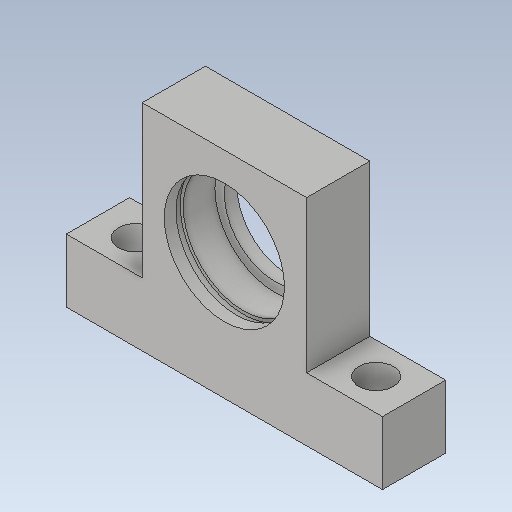
# Autodesk Inventor part: BGHK6800VV-20_h
Saved by Autodesk Inventor 2020.2 (Build 242310000, 310)
## iProperties
Created: 2022-11-02
Part Number: BGHK6800VV-20_h
Material: Generic
Catalog Web Link: www.cadenas.de
Description: BGHKB, BGHK, BGHKA, BGHKSA, BGHKS_housing-Bearings with Housings - T-Shaped - h Selectable
Vendor: MISUMI
Document SubType Name: Modeling
Designer: psAdmin
Manufacturer: MISUMI
Mass: 8.05926 g
Surface Area: 44.1935 cm^2
Volume: 8.05926 cm^3
Density: 1 g/cm^3
Appearance: PSOLRGB-175-175-175
Category: PARTsolutions
Company: MISUMI
PSOL_IDENT_0: {$CADENAS_DATA/23d-libs/misumi/metric/12_bearing_holders/bghkb/bghkb_housing.prj},237 {VTYP=3D},{NB=
PSOL_IDENT_1: BGHK6800VV-20_h},{LINA=BGHK6800VV-20},{NN=BGHKB, BGHK, BGHKA, BGHKSA, BGHKS_housing},{DATE=30.03.201
PSOL_IDENT_2: 8 01:48:21},{GEOMDATE=23.03.2015 00:00:00},{VERSION=},{LINEID=300},{WBVAR=MATB,MATH,STH,SEAL,HH,ALT1
PSOL_IDENT_3: ,ALT2},{WBNUMERIC=HH}  {NB=BGHK6800VV-20_h},{LINA=BGHK6800VV-20},{KT=DUMMY},{PN=BGHK6800VV-20},{TYPE=
PSOL_IDENT_4: BGHK},{MATB=S},{MATBALG='S','Steel','SS','Stainless Steel'},{MATH=S45C},{MATHALG='S45C','1045 Carbon
PSOL_IDENT_5: Steel','2017AA','2017 Aluminum Alloy'},{STH=ENP},{STHALG='BO','Black Oxide','ENP','Electroless Nick
PSOL_IDENT_6: el Plating'},{ARR=304 Stainless Steel},{ARR3D=-S},{BN=6800},{SEAL=VV},{SEALALG='ZZ','Double Shielded'
PSOL_IDENT_7: ,'VV','Non-Contact Sealed Rubber Seal','DD','Contact Sealed Rubber Seal'},{HH=20},{HHALG=[20,25,30]}
PSOL_IDENT_8: ,{DD=10},{D=19},{DD2=20},{MM=1.15},{DDHH=16},{B=5},{LL1=2},{H=34},{H2=14},{L=50},{L1=38.0},{L2=26},{
PSOL_IDENT_9: T=10},{S=10},{DD1=5.5},{ALT1=},{ALT2=}
NB: BGHK6800VV-20_h
NN: BGHKB, BGHK, BGHKA, BGHKSA, BGHKS_housing
NT: Bearings with Housings - T-Shaped - h Selectable
NBSYN: $PN._h
LINA: BGHK6800VV-20
CATALOG: Misumi
PN: BGHK6800VV-20
MATB: Steel
MATH: 1045 Carbon Steel
STH: Electroless Nickel Plating
ARR: 304 Stainless Steel
BN: 6800
SEAL: Non-Contact Sealed Rubber Seal
HH: 20
DD: 10
D: 19
DDHH: 16
B: 5
LL1: 2
H: 34
L: 50
L1: 38
L2: 26
T: 10
S: 10
DD1: 5.5
ALT1: Bearings, Retaining Rings Assembled
ALT2: w/o KCC (C2 Chamfer)
SUPPLIER: MISUMI
ARTICLENO: BGHK6800VV-20_h
BOMINFO: BGHK6800VV-20
CREATOR: CADENAS GmbH
Title: BGHK6800VV-20
Author: Cadenas PARTsolutions
Comments: Bearings with Housings - T-Shaped - h Selectable
Autodesk Inventor part; units mm, degrees
sketch "Sketch_1" plane through (0, 0, 0) normal (0, 0, 1) x (1, 0, 0)
  line L0 (-25, -10) -> (-25, -20)
  line L1 (-25, -20) -> (25, -20)
  line L2 (25, -20) -> (25, -10)
  line L3 (25, -10) -> (13, -10)
  line L4 (13, -10) -> (13, 14)
  line L5 (13, 14) -> (-13, 14)
  line L6 (-13, 14) -> (-13, -10)
  line L7 (-13, -10) -> (-25, -10)
  constraints: 16 end point
extrude "Extrusion1" add sketch "Sketch_1" along normal mid plane 10
sketch "Sketch2" plane through (0, 0, 5) normal (0, 0, 1) x (1, 0, 0)
  point P0 (0, 0)
hole "Hole1" at (0, 0, 5) direction (0, 0, -1) diameter 16 depth 10 counterbore diameter 19 counterbore depth 8
sketch "Sketch3" plane through (-25, -20, 5) normal (0, -1, 0) x (1, 0, 0)
  point P0 (6, -5)
hole "Hole2" at (-19, -20, 0) direction (0, 1, 0) diameter 5.5 depth 10
sketch "Sketch4" plane through (-25, -20, 5) normal (0, -1, 0) x (1, 0, 0)
  point P0 (44, -5)
hole "Hole3" at (19, -20, 0) direction (0, 1, 0) diameter 5.5 depth 10
sketch "Sketch_4" plane through (0, 0, 0) normal (1, 0, 0) x (0, 0, -1)
  line L0 (-2, 0) -> (-3.15, 0)
  line L1 (-3.15, 0) -> (-3.15, 10)
  line L2 (-3.15, 10) -> (-2, 10)
  line L3 (-2, 10) -> (-2, 0)
  line L4 (-2, 0) -> (-3.15, 0)
  constraints: 10 end point
revolve "Revolution1" cut sketch "Sketch_4" angle 360 about axis through (0, 0, 2) along (0, 0, -1)
ref_plane "housing_to_dummy_XY" through (0, 0, 0) normal (1, 0, 0) x (0, 0, -1)
ref_plane "housing_to_dummy_YZ" through (0, 0, 0) normal (0, 0, -1) x (0, 1, 0)
ref_plane "housing_to_dummy_ZX" through (0, 0, 0) normal (0, 1, 0) x (1, 0, 0)
ref_plane "to_bearing_XY" through (0, 0, -3) normal (0, 0, -1) x (1, 0, 0)
ref_plane "to_bearing_YZ" through (0, 0, -3) normal (1, 0, 0) x (0, -1, 0)
ref_plane "to_bearing_ZX" through (0, 0, -3) normal (0, -1, 0) x (0, 0, -1)
ref_plane "to_rring_XY" through (0, 0, 2) normal (0, 0, -1) x (1, 0, 0)
ref_plane "to_rring_YZ" through (0, 0, 2) normal (1, 0, 0) x (0, -1, 0)
ref_plane "to_rring_ZX" through (0, 0, 2) normal (0, -1, 0) x (0, 0, -1)
body "Solid1"
